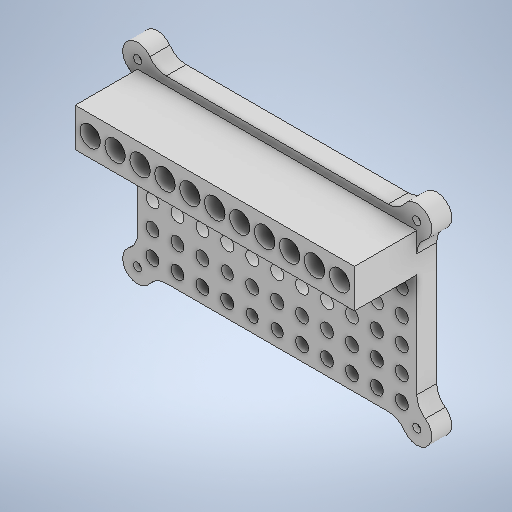
# Autodesk Inventor part: Top_Tip_Matrix
Saved by Autodesk Inventor 2025.2 (Build 292293000, 293)
## iProperties
Created: 2025-02-14
Part Number: Top_Tip_Matrix
Material: Generic
Document SubType Name: Modeling
Designer: m_kni
Density: 1 g/cm^3
Appearance: Default
Author: m_kni
## iProperties of the stored document Top_Tip_Matrix_3DPrint.ipt
Created: 2025-02-16
Part Number: Top_Tip_Matrix_3DPrint
Material: Generic
Document SubType Name: Modeling
Designer: m_kni
Density: 1 g/cm^3
Appearance: Default
Author: m_kni
Autodesk Inventor part; units mm, degrees
ref_plane "YZ Plane" through (0, 0, 0) normal (1, 0, 0) x (0, 1, 0)
ref_plane "XZ Plane" through (0, 0, 0) normal (0, 1, 0) x (-1, 0, 0)
ref_plane "XY Plane" through (0, 0, 0) normal (0, 0, 1) x (1, 0, 0)
sketch "Sketch1" plane through (0, 0, 0) normal (0, 0, 1) x (1, 0, 0)
  line L0 (55, -36) -> (-55, -36)
  line L1 (-55, -36) -> (-55, 36)
  line L2 (-55, 36) -> (55, 36)
  line L3 (55, -36) -> (-55, 36) construction
  line L4 (-55, -36) -> (55, 36) construction
  circle A0 centre (-49, 30) radius 2.425
  circle A1 centre (-49, 20) radius 2.425
  circle A2 centre (-49, 10) radius 2.425
  circle A3 centre (-49, 0) radius 2.425
  circle A4 centre (-49, -10) radius 2.425
  circle A5 centre (-49, -20) radius 2.425
  circle A6 centre (-49, -30) radius 2.425
  circle A7 centre (-39, 30) radius 2.425
  circle A8 centre (-39, 20) radius 2.425
  circle A9 centre (-39, 10) radius 2.425
  circle A10 centre (-39, 0) radius 2.425
  circle A11 centre (-39, -10) radius 2.425
  circle A12 centre (-39, -20) radius 2.425
  circle A13 centre (-39, -30) radius 2.425
  circle A14 centre (-29, 30) radius 2.425
  circle A15 centre (-29, 20) radius 2.425
  circle A16 centre (-29, 10) radius 2.425
  circle A17 centre (-29, 0) radius 2.425
  circle A18 centre (-29, -10) radius 2.425
  circle A19 centre (-29, -20) radius 2.425
  circle A20 centre (-29, -30) radius 2.425
  circle A21 centre (-19, 30) radius 2.425
  circle A22 centre (-19, 20) radius 2.425
  circle A23 centre (-19, 10) radius 2.425
  circle A24 centre (-19, 0) radius 2.425
  circle A25 centre (-19, -10) radius 2.425
  circle A26 centre (-19, -20) radius 2.425
  circle A27 centre (-19, -30) radius 2.425
  circle A28 centre (-9, 30) radius 2.425
  circle A29 centre (-9, 20) radius 2.425
  circle A30 centre (-9, 10) radius 2.425
  circle A31 centre (-9, 0) radius 2.425
  circle A32 centre (-9, -10) radius 2.425
  circle A33 centre (-9, -20) radius 2.425
  circle A34 centre (-9, -30) radius 2.425
  circle A35 centre (1, 30) radius 2.425
  circle A36 centre (1, 20) radius 2.425
  circle A37 centre (1, 10) radius 2.425
  circle A38 centre (1, 0) radius 2.425
  circle A39 centre (1, -10) radius 2.425
  circle A40 centre (1, -20) radius 2.425
  circle A41 centre (1, -30) radius 2.425
  circle A42 centre (11, 30) radius 2.425
  circle A43 centre (11, 20) radius 2.425
  circle A44 centre (11, 10) radius 2.425
  circle A45 centre (11, 0) radius 2.425
  circle A46 centre (11, -10) radius 2.425
  circle A47 centre (11, -20) radius 2.425
  circle A48 centre (11, -30) radius 2.425
  circle A49 centre (21, 30) radius 2.425
  circle A50 centre (21, 20) radius 2.425
  circle A51 centre (21, 10) radius 2.425
  circle A52 centre (21, 0) radius 2.425
  circle A53 centre (21, -10) radius 2.425
  circle A54 centre (21, -20) radius 2.425
  circle A55 centre (21, -30) radius 2.425
  circle A56 centre (31, 30) radius 2.425
  circle A57 centre (31, 20) radius 2.425
  circle A58 centre (31, 10) radius 2.425
  circle A59 centre (31, 0) radius 2.425
  circle A60 centre (31, -10) radius 2.425
  circle A61 centre (31, -20) radius 2.425
  circle A62 centre (31, -30) radius 2.425
  circle A63 centre (41, 30) radius 2.425
  circle A64 centre (41, 20) radius 2.425
  circle A65 centre (41, 10) radius 2.425
  circle A66 centre (41, 0) radius 2.425
  circle A67 centre (41, -10) radius 2.425
  circle A68 centre (41, -20) radius 2.425
  circle A69 centre (41, -30) radius 2.425
  circle A70 centre (51, 30) radius 2.425
  circle A71 centre (51, 20) radius 2.425
  circle A72 centre (51, 10) radius 2.425
  circle A73 centre (51, 0) radius 2.425
  circle A74 centre (51, -10) radius 2.425
  circle A75 centre (51, -20) radius 2.425
  circle A76 centre (51, -30) radius 2.425
  line L5 (-55, 36) -> (57, 36)
  line L6 (57, 36) -> (57, -36)
  line L7 (57, -36) -> (-55, -36)
  line L8 (-55, -36) -> (-55, 36)
  circle A77 centre (-55, 36) radius 6
  circle A78 centre (-55, -36) radius 6
  circle A79 centre (57, 36) radius 6
  circle A80 centre (57, -36) radius 6
  point P0 (0, 0)
  point P1 (57, 30)
  point P2 (-49, -36)
  point P3 (57, -30)
  point P4 (57, 30)
  point P5 (51, 36)
  point P6 (-49, 36)
  point P7 (-55, 30)
  point P8 (-55, -30)
  point P9 (-49, -36)
  point P10 (51, -36)
  dimension "d0" = 110
  dimension "d1" = 72
  dimension "d2" = 4.85
  dimension "d3" = 6
  dimension "d4" = 6
  dimension "d7" = 10
  dimension "d10" = 10
  dimension "d13" = 6
  dimension "d14" = 6
  dimension "d15" = 12
  dimension "d16" = 12
  dimension "d17" = 12
  dimension "d18" = 12
  constraints: 81 centre point, 18 end point, 5 coincident, 3 horizontal, 3 parallel, 2 midpoint, 2 perpendicular, 1 vertical, 152 other
  measures "d0" distance of L1.end L2.end
  measures "d1" distance of L0.end L1.end
  measures "d2" diameter of A0
  measures "d3" distance from line of A0.centre L2
  measures "d4" distance from line of A0.centre L1
  measures "d7" distance of A0.centre A1.centre
  measures "d10" distance of A0.centre A7.centre
  measures "d13" distance of point (57, 30) A70.centre
  measures "d14" distance of point (-49, -36) A6.centre
  measures "d15" diameter of A77
  measures "d16" diameter of A78
  measures "d17" diameter of A79
  measures "d18" diameter of A80
extrude "Extrusion1" add sketch "Sketch1" along normal blind 8
sketch "Sketch2" plane through (0, 0, 8) normal (0, 0, 1) x (1, 0, 0)
  arc A0 (-49, 36) -> (-55, 30) centre (-55, 36) ccw projected
  arc A1 (57, 30) -> (51, 36) centre (57, 36) ccw projected
  line L0 (51, 36) -> (-49, 36) projected
  arc A2 (-49, 36) -> (-55, 30) centre (-55, 36) ccw projected
  line L1 (-55, 30) -> (-55, -30) projected
  arc A3 (-55, -30) -> (-49, -36) centre (-55, -36) ccw projected
  line L2 (-49, -36) -> (51, -36) projected
  arc A4 (51, -36) -> (57, -30) centre (57, -36) ccw projected
  line L3 (57, -30) -> (57, 30) projected
  circle A5 centre (51, -10) radius 2.425 projected
  circle A6 centre (51, 10) radius 2.425 projected
  circle A7 centre (41, -30) radius 2.425 projected
  circle A8 centre (41, -10) radius 2.425 projected
  circle A9 centre (41, 10) radius 2.425 projected
  circle A10 centre (41, 30) radius 2.425 projected
  circle A11 centre (31, -20) radius 2.425 projected
  circle A12 centre (31, 0) radius 2.425 projected
  circle A13 centre (31, 20) radius 2.425 projected
  circle A14 centre (21, -30) radius 2.425 projected
  circle A15 centre (21, -10) radius 2.425 projected
  circle A16 centre (21, 10) radius 2.425 projected
  circle A17 centre (21, 30) radius 2.425 projected
  circle A18 centre (11, -20) radius 2.425 projected
  circle A19 centre (11, 0) radius 2.425 projected
  circle A20 centre (11, 20) radius 2.425 projected
  circle A21 centre (1, -30) radius 2.425 projected
  circle A22 centre (1, -10) radius 2.425 projected
  circle A23 centre (1, 10) radius 2.425 projected
  circle A24 centre (1, 30) radius 2.425 projected
  circle A25 centre (-9, -20) radius 2.425 projected
  circle A26 centre (-9, 0) radius 2.425 projected
  circle A27 centre (-9, 20) radius 2.425 projected
  circle A28 centre (-19, -30) radius 2.425 projected
  circle A29 centre (-19, -10) radius 2.425 projected
  circle A30 centre (-19, 10) radius 2.425 projected
  circle A31 centre (-19, 30) radius 2.425 projected
  circle A32 centre (-29, -20) radius 2.425 projected
  circle A33 centre (-29, 0) radius 2.425 projected
  circle A34 centre (-29, 20) radius 2.425 projected
  circle A35 centre (-39, -30) radius 2.425 projected
  circle A36 centre (-39, -10) radius 2.425 projected
  circle A37 centre (-39, 10) radius 2.425 projected
  circle A38 centre (-49, 20) radius 2.425 projected
  circle A39 centre (-49, 10) radius 2.425 projected
  circle A40 centre (-49, 0) radius 2.425 projected
  circle A41 centre (-49, -10) radius 2.425 projected
  circle A42 centre (-49, -20) radius 2.425 projected
  circle A43 centre (-39, 30) radius 2.425 projected
  circle A44 centre (-39, 20) radius 2.425 projected
  circle A45 centre (-39, 0) radius 2.425 projected
  circle A46 centre (-39, -20) radius 2.425 projected
  circle A47 centre (-29, 30) radius 2.425 projected
  circle A48 centre (-29, 10) radius 2.425 projected
  circle A49 centre (-29, -10) radius 2.425 projected
  circle A50 centre (-29, -30) radius 2.425 projected
  circle A51 centre (-19, 20) radius 2.425 projected
  circle A52 centre (-19, 0) radius 2.425 projected
  circle A53 centre (-19, -20) radius 2.425 projected
  circle A54 centre (-9, 30) radius 2.425 projected
  circle A55 centre (-9, 10) radius 2.425 projected
  circle A56 centre (-9, -10) radius 2.425 projected
  circle A57 centre (-9, -30) radius 2.425 projected
  circle A58 centre (1, 20) radius 2.425 projected
  circle A59 centre (1, 0) radius 2.425 projected
  circle A60 centre (1, -20) radius 2.425 projected
  circle A61 centre (11, 30) radius 2.425 projected
  circle A62 centre (11, 10) radius 2.425 projected
  circle A63 centre (11, -10) radius 2.425 projected
  circle A64 centre (11, -30) radius 2.425 projected
  circle A65 centre (21, 20) radius 2.425 projected
  circle A66 centre (21, 0) radius 2.425 projected
  circle A67 centre (21, -20) radius 2.425 projected
  circle A68 centre (31, 30) radius 2.425 projected
  circle A69 centre (31, 10) radius 2.425 projected
  circle A70 centre (31, -10) radius 2.425 projected
  circle A71 centre (31, -30) radius 2.425 projected
  circle A72 centre (41, 20) radius 2.425 projected
  circle A73 centre (41, 0) radius 2.425 projected
  circle A74 centre (41, -20) radius 2.425 projected
  circle A75 centre (51, 20) radius 2.425 projected
  circle A76 centre (51, 0) radius 2.425 projected
  circle A77 centre (51, -20) radius 2.425 projected
  circle A78 centre (51, -30) radius 2.425 projected
  circle A79 centre (51, 30) radius 2.425 projected
  circle A80 centre (-49, -30) radius 2.425 projected
  circle A81 centre (-49, 30) radius 2.425 projected
  circle A82 centre (-55, 36) radius 4
  circle A83 centre (-55, -36) radius 4
  circle A84 centre (57, -36) radius 4
  circle A85 centre (57, 36) radius 4
  circle A86 centre (-49, 30) radius 2.6
  circle A87 centre (-39, 30) radius 2.6
  circle A88 centre (-29, 30) radius 2.6
  circle A89 centre (-19, 30) radius 2.6
  circle A90 centre (-9, 30) radius 2.6
  circle A91 centre (1, 30) radius 2.6
  circle A92 centre (11, 30) radius 2.6
  circle A93 centre (21, 30) radius 2.6
  circle A94 centre (31, 30) radius 2.6
  circle A95 centre (41, 30) radius 2.6
  circle A96 centre (51, 30) radius 2.6
  circle A97 centre (-49, 20) radius 2.6
  circle A98 centre (-39, 20) radius 2.6
  circle A99 centre (-29, 20) radius 2.6
  circle A100 centre (-19, 20) radius 2.6
  circle A101 centre (-9, 20) radius 2.6
  circle A102 centre (1, 20) radius 2.6
  circle A103 centre (11, 20) radius 2.6
  circle A104 centre (21, 20) radius 2.6
  circle A105 centre (31, 20) radius 2.6
  circle A106 centre (41, 20) radius 2.6
  circle A107 centre (51, 20) radius 2.6
  circle A108 centre (-49, 10) radius 2.6
  circle A109 centre (-39, 10) radius 2.6
  circle A110 centre (-29, 10) radius 2.6
  circle A111 centre (-19, 10) radius 2.6
  circle A112 centre (-9, 10) radius 2.6
  circle A113 centre (1, 10) radius 2.6
  circle A114 centre (11, 10) radius 2.6
  circle A115 centre (21, 10) radius 2.6
  circle A116 centre (31, 10) radius 2.6
  circle A117 centre (41, 10) radius 2.6
  circle A118 centre (51, 10) radius 2.6
  circle A119 centre (-49, 0) radius 2.6
  circle A120 centre (-39, 0) radius 2.6
  circle A121 centre (-29, 0) radius 2.6
  circle A122 centre (-19, 0) radius 2.6
  circle A123 centre (-9, 0) radius 2.6
  circle A124 centre (1, 0) radius 2.6
  circle A125 centre (11, 0) radius 2.6
  circle A126 centre (21, 0) radius 2.6
  circle A127 centre (31, 0) radius 2.6
  circle A128 centre (41, 0) radius 2.6
  circle A129 centre (51, 0) radius 2.6
  circle A130 centre (-49, -10) radius 2.6
  circle A131 centre (-39, -10) radius 2.6
  circle A132 centre (-29, -10) radius 2.6
  circle A133 centre (-19, -10) radius 2.6
  circle A134 centre (-9, -10) radius 2.6
  circle A135 centre (1, -10) radius 2.6
  circle A136 centre (11, -10) radius 2.6
  circle A137 centre (21, -10) radius 2.6
  circle A138 centre (31, -10) radius 2.6
  circle A139 centre (41, -10) radius 2.6
  circle A140 centre (51, -10) radius 2.6
  circle A141 centre (-49, -20) radius 2.6
  circle A142 centre (-39, -20) radius 2.6
  circle A143 centre (-29, -20) radius 2.6
  circle A144 centre (-19, -20) radius 2.6
  circle A145 centre (-9, -20) radius 2.6
  circle A146 centre (1, -20) radius 2.6
  circle A147 centre (11, -20) radius 2.6
  circle A148 centre (21, -20) radius 2.6
  circle A149 centre (31, -20) radius 2.6
  circle A150 centre (41, -20) radius 2.6
  circle A151 centre (51, -20) radius 2.6
  circle A152 centre (-49, -30) radius 2.6
  circle A153 centre (-39, -30) radius 2.6
  circle A154 centre (-29, -30) radius 2.6
  circle A155 centre (-19, -30) radius 2.6
  circle A156 centre (-9, -30) radius 2.6
  circle A157 centre (1, -30) radius 2.6
  circle A158 centre (11, -30) radius 2.6
  circle A159 centre (21, -30) radius 2.6
  circle A160 centre (31, -30) radius 2.6
  circle A161 centre (41, -30) radius 2.6
  circle A162 centre (51, -30) radius 2.6
  point P0 (0, 0)
  dimension "d21" = 8
  dimension "d22" = 8
  dimension "d23" = 8
  dimension "d24" = 8
  dimension "d36" = 4.85
  dimension "d37" = 5.2
  dimension "d40" = 10
  dimension "d43" = 10
  constraints: 81 centre point, 5 coincident, 1 horizontal, 1 vertical, 152 other
  measures "d21" diameter of A82
  measures "d22" diameter of A83
  measures "d23" diameter of A84
  measures "d24" diameter of A85
  measures "d36" diameter of A64
  measures "d37" diameter of A86
  measures "d40" distance of A86.centre A87.centre
  measures "d43" distance of A86.centre A97.centre
extrude "Extrusion2" cut sketch "Sketch2" against normal blind 8 contours A82 | A83 | A84 | A85
sketch "Sketch3" plane through (0, 0, 8) normal (0, 0, 1) x (1, 0, 0)
  circle A0 centre (-55, 36) radius 4 projected
  circle A1 centre (-55, -36) radius 4 projected
  circle A2 centre (57, 36) radius 4 projected
  circle A3 centre (57, -36) radius 4 projected
  point P0 (0, 0)
extrude "Extrusion3" add sketch "Sketch3" against normal blind 2
sketch "Sketch4" plane through (0, 0, 8) normal (0, 0, 1) x (1, 0, 0)
  arc A0 (-49, 36) -> (-55, 30) centre (-55, 36) ccw projected
  arc A1 (57, 30) -> (51, 36) centre (57, 36) ccw projected
  arc A2 (-55, -30) -> (-49, -36) centre (-55, -36) ccw projected
  arc A3 (51, -36) -> (57, -30) centre (57, -36) ccw projected
  circle A4 centre (-55, 36) radius 1.6
  circle A5 centre (-55, -36) radius 4 projected
  circle A6 centre (-55, -36) radius 1.6
  circle A7 centre (57, 36) radius 1.6
  circle A8 centre (57, -36) radius 1.6
  point P0 (0, 0)
  dimension "d29" = 3.2
  dimension "d30" = 3.2
  dimension "d31" = 3.2
  dimension "d32" = 3.2
  constraints: 4 centre point, 4 coincident
  measures "d29" diameter of A4
  measures "d30" diameter of A6
  measures "d31" diameter of A7
  measures "d32" diameter of A8
extrude "Extrusion4" cut sketch "Sketch4" against normal blind 22.6375 contours A4 | A6 | A7 | A8
fillet "Fillet1" radius 8 8 edges at (-49, 36, 4) (51, 36, 4) (57, 30, 4) (57, -30, 4) (51, -36, 4) (-49, -36, 4) (-55, -30, 4) (-55, 30, 4)
sketch "Sketch5" plane through (0, 0, 0) normal (0, 0, -1) x (-1, 0, 0)
  circle A0 centre (49, 30) radius 2.425 projected
  circle A1 centre (39, 30) radius 2.425 projected
  circle A2 centre (-57, -36) radius 4 projected
  circle A3 centre (55, -36) radius 4 projected
  circle A4 centre (-57, 36) radius 4 projected
  circle A5 centre (55, 36) radius 4 projected
  arc A6 (-57, 24.5109) -> (-60.4286, 31.0761) centre (-65, 24.5109) ccw projected
  line L0 (-57, -24.5109) -> (-57, 24.5109) projected
  arc A7 (-60.4286, -31.0761) -> (-57, -24.5109) centre (-65, -24.5109) ccw projected
  arc A8 (-60.4286, -31.0761) -> (-52.0761, -39.4286) centre (-57, -36) ccw projected
  arc A9 (-45.5109, -36) -> (-52.0761, -39.4286) centre (-45.5109, -44) ccw projected
  line L1 (43.5109, -36) -> (-45.5109, -36) projected
  arc A10 (50.0761, -39.4286) -> (43.5109, -36) centre (43.5109, -44) ccw projected
  arc A11 (50.0761, -39.4286) -> (58.4286, -31.0761) centre (55, -36) ccw projected
  arc A12 (55, -24.5109) -> (58.4286, -31.0761) centre (63, -24.5109) ccw projected
  line L2 (55, 24.5109) -> (55, -24.5109) projected
  arc A13 (58.4286, 31.0761) -> (55, 24.5109) centre (63, 24.5109) ccw projected
  arc A14 (58.4286, 31.0761) -> (50.0761, 39.4286) centre (55, 36) ccw projected
  arc A15 (43.5109, 36) -> (50.0761, 39.4286) centre (43.5109, 44) ccw projected
  line L3 (-45.5109, 36) -> (43.5109, 36) projected
  arc A16 (-52.0761, 39.4286) -> (-45.5109, 36) centre (-45.5109, 44) ccw projected
  arc A17 (-52.0761, 39.4286) -> (-60.4286, 31.0761) centre (-57, 36) ccw projected
  circle A18 centre (-51, -10) radius 2.425 projected
  circle A19 centre (-51, 10) radius 2.425 projected
  circle A20 centre (-41, -30) radius 2.425 projected
  circle A21 centre (-41, -10) radius 2.425 projected
  circle A22 centre (-41, 10) radius 2.425 projected
  circle A23 centre (-41, 30) radius 2.425 projected
  circle A24 centre (-31, -20) radius 2.425 projected
  circle A25 centre (-31, 0) radius 2.425 projected
  circle A26 centre (-31, 20) radius 2.425 projected
  circle A27 centre (-21, -30) radius 2.425 projected
  circle A28 centre (-21, -10) radius 2.425 projected
  circle A29 centre (-21, 10) radius 2.425 projected
  circle A30 centre (-21, 30) radius 2.425 projected
  circle A31 centre (-11, -20) radius 2.425 projected
  circle A32 centre (-11, 0) radius 2.425 projected
  circle A33 centre (-11, 20) radius 2.425 projected
  circle A34 centre (-1, -30) radius 2.425 projected
  circle A35 centre (-1, -10) radius 2.425 projected
  circle A36 centre (-1, 10) radius 2.425 projected
  circle A37 centre (-1, 30) radius 2.425 projected
  circle A38 centre (9, -20) radius 2.425 projected
  circle A39 centre (9, 0) radius 2.425 projected
  circle A40 centre (9, 20) radius 2.425 projected
  circle A41 centre (19, -30) radius 2.425 projected
  circle A42 centre (19, -10) radius 2.425 projected
  circle A43 centre (19, 10) radius 2.425 projected
  circle A44 centre (19, 30) radius 2.425 projected
  circle A45 centre (29, -20) radius 2.425 projected
  circle A46 centre (29, 0) radius 2.425 projected
  circle A47 centre (29, 20) radius 2.425 projected
  circle A48 centre (39, -30) radius 2.425 projected
  circle A49 centre (39, -10) radius 2.425 projected
  circle A50 centre (39, 10) radius 2.425 projected
  circle A51 centre (49, 20) radius 2.425 projected
  circle A52 centre (49, 10) radius 2.425 projected
  circle A53 centre (49, 0) radius 2.425 projected
  circle A54 centre (49, -10) radius 2.425 projected
  circle A55 centre (49, -20) radius 2.425 projected
  circle A56 centre (39, 30) radius 2.425 projected
  circle A57 centre (39, 20) radius 2.425 projected
  circle A58 centre (39, 0) radius 2.425 projected
  circle A59 centre (39, -20) radius 2.425 projected
  circle A60 centre (29, 30) radius 2.425 projected
  circle A61 centre (29, 10) radius 2.425 projected
  circle A62 centre (29, -10) radius 2.425 projected
  circle A63 centre (29, -30) radius 2.425 projected
  circle A64 centre (19, 20) radius 2.425 projected
  circle A65 centre (19, 0) radius 2.425 projected
  circle A66 centre (19, -20) radius 2.425 projected
  circle A67 centre (9, 30) radius 2.425 projected
  circle A68 centre (9, 10) radius 2.425 projected
  circle A69 centre (9, -10) radius 2.425 projected
  circle A70 centre (9, -30) radius 2.425 projected
  circle A71 centre (-1, 20) radius 2.425 projected
  circle A72 centre (-1, 0) radius 2.425 projected
  circle A73 centre (-1, -20) radius 2.425 projected
  circle A74 centre (-11, 30) radius 2.425 projected
  circle A75 centre (-11, 10) radius 2.425 projected
  circle A76 centre (-11, -10) radius 2.425 projected
  circle A77 centre (-11, -30) radius 2.425 projected
  circle A78 centre (-21, 20) radius 2.425 projected
  circle A79 centre (-21, 0) radius 2.425 projected
  circle A80 centre (-21, -20) radius 2.425 projected
  circle A81 centre (-31, 30) radius 2.425 projected
  circle A82 centre (-31, 10) radius 2.425 projected
  circle A83 centre (-31, -10) radius 2.425 projected
  circle A84 centre (-31, -30) radius 2.425 projected
  circle A85 centre (-41, 20) radius 2.425 projected
  circle A86 centre (-41, 0) radius 2.425 projected
  circle A87 centre (-41, -20) radius 2.425 projected
  circle A88 centre (-51, 20) radius 2.425 projected
  circle A89 centre (-51, 0) radius 2.425 projected
  circle A90 centre (-51, -20) radius 2.425 projected
  circle A91 centre (-51, -30) radius 2.425 projected
  circle A92 centre (-51, 30) radius 2.425 projected
  circle A93 centre (49, -30) radius 2.425 projected
  circle A94 centre (49, 30) radius 2.425 projected
  circle A95 centre (29, 30) radius 2.425 projected
  circle A96 centre (49, 30) radius 2.625
  circle A97 centre (49, 20) radius 2.625
  circle A98 centre (49, 10) radius 2.625
  circle A99 centre (49, 0) radius 2.625
  circle A100 centre (49, -10) radius 2.625
  circle A101 centre (49, -20) radius 2.625
  circle A102 centre (49, -30) radius 2.625
  circle A103 centre (39, 30) radius 2.625
  circle A104 centre (39, 20) radius 2.625
  circle A105 centre (39, 10) radius 2.625
  circle A106 centre (39, 0) radius 2.625
  circle A107 centre (39, -10) radius 2.625
  circle A108 centre (39, -20) radius 2.625
  circle A109 centre (39, -30) radius 2.625
  circle A110 centre (29, 30) radius 2.625
  circle A111 centre (29, 20) radius 2.625
  circle A112 centre (29, 10) radius 2.625
  circle A113 centre (29, 0) radius 2.625
  circle A114 centre (29, -10) radius 2.625
  circle A115 centre (29, -20) radius 2.625
  circle A116 centre (29, -30) radius 2.625
  circle A117 centre (19, 30) radius 2.625
  circle A118 centre (19, 20) radius 2.625
  circle A119 centre (19, 10) radius 2.625
  circle A120 centre (19, 0) radius 2.625
  circle A121 centre (19, -10) radius 2.625
  circle A122 centre (19, -20) radius 2.625
  circle A123 centre (19, -30) radius 2.625
  circle A124 centre (9, 30) radius 2.625
  circle A125 centre (9, 20) radius 2.625
  circle A126 centre (9, 10) radius 2.625
  circle A127 centre (9, 0) radius 2.625
  circle A128 centre (9, -10) radius 2.625
  circle A129 centre (9, -20) radius 2.625
  circle A130 centre (9, -30) radius 2.625
  circle A131 centre (-1, 30) radius 2.625
  circle A132 centre (-1, 20) radius 2.625
  circle A133 centre (-1, 10) radius 2.625
  circle A134 centre (-1, 0) radius 2.625
  circle A135 centre (-1, -10) radius 2.625
  circle A136 centre (-1, -20) radius 2.625
  circle A137 centre (-1, -30) radius 2.625
  circle A138 centre (-11, 30) radius 2.625
  circle A139 centre (-11, 20) radius 2.625
  circle A140 centre (-11, 10) radius 2.625
  circle A141 centre (-11, 0) radius 2.625
  circle A142 centre (-11, -10) radius 2.625
  circle A143 centre (-11, -20) radius 2.625
  circle A144 centre (-11, -30) radius 2.625
  circle A145 centre (-21, 30) radius 2.625
  circle A146 centre (-21, 20) radius 2.625
  circle A147 centre (-21, 10) radius 2.625
  circle A148 centre (-21, 0) radius 2.625
  circle A149 centre (-21, -10) radius 2.625
  circle A150 centre (-21, -20) radius 2.625
  circle A151 centre (-21, -30) radius 2.625
  circle A152 centre (-31, 30) radius 2.625
  circle A153 centre (-31, 20) radius 2.625
  circle A154 centre (-31, 10) radius 2.625
  circle A155 centre (-31, 0) radius 2.625
  circle A156 centre (-31, -10) radius 2.625
  circle A157 centre (-31, -20) radius 2.625
  circle A158 centre (-31, -30) radius 2.625
  circle A159 centre (-41, 30) radius 2.625
  circle A160 centre (-41, 20) radius 2.625
  circle A161 centre (-41, 10) radius 2.625
  circle A162 centre (-41, 0) radius 2.625
  circle A163 centre (-41, -10) radius 2.625
  circle A164 centre (-41, -20) radius 2.625
  circle A165 centre (-41, -30) radius 2.625
  circle A166 centre (-51, 30) radius 2.625
  circle A167 centre (-51, 20) radius 2.625
  circle A168 centre (-51, 10) radius 2.625
  circle A169 centre (-51, 0) radius 2.625
  circle A170 centre (-51, -10) radius 2.625
  circle A171 centre (-51, -20) radius 2.625
  circle A172 centre (-51, -30) radius 2.625
  point P0 (0, 0)
  dimension "d46" = 5.25
  dimension "d49" = 10
  dimension "d52" = 10
  constraints: 77 centre point, 1 coincident, 1 horizontal, 1 vertical, 152 other
  measures "d46" diameter of A96
  measures "d49" distance of A96.centre A97.centre
  measures "d52" distance of A96.centre A103.centre
extrude "Extrusion5" cut sketch "Sketch5" against normal blind 10 contours A0 | A1 | A18 | A19 | A20 | A21 | A22 | A23 | A24 | A25 | A26 | A27 | A28 | A29 | A30 | A31 | A32 | A33 | A34 | A35 | A36 | A37 | A38 | A39 | A40 | A41 | A42 | A43 | A44 | A45 | A46 | A47 | A48 | A49 | A50 | A51 | A52 | A53 | A54 | A55 | A57 | A58 | A59 | A60 | A61 | A62 | A63 | A64 | A65 | A66 | A67 | A68 | A69 | A70 | A71 | A72 | A73 | A74 | A75 | A76 | A77 | A78 | A79 | A80 | A81 | A82 | A83 | A84 | A85 | A86 | A87 | A88 | A89 | A90 | A91 | A92 | A93 | A96 | A97 | A98 | A99 | A100 | A101 | A102 | A103 | A104 | A105 | A106 | A107 | A108 | A109 | A110 | A111 | A112 | A113 | A114 | A115 | A116 | A117 | A118 | A119 | A120 | A121 | A123 | A124 | A125 | A126 | A127 | A128 | A129 | A131 | A132 | A133 | A134 | A135 | A136 | A138 | A139 | A140 | A141 | A142 | A143 | A144 | A145 | A146 | A147 | A148 | A149 | A150 | A151 | A152 | A153 | A154 | A155 | A156 | A157 | A158 | A159 | A160 | A161 | A162 | A163 | A164 | A165 | A166 | A167 | A168 | A169 | A170 | A171 | A172
sketch "Sketch7" plane through (0, 0, 8) normal (0, 0, 1) x (1, 0, 0)
  line L0 (-55, 24.5109) -> (-55, -24.5109) projected
  line L1 (-55, 17.1851) -> (57, 17.1851)
  line L2 (57, -24.5109) -> (57, 24.5109) projected
  line L3 (-55, 17.1851) -> (53.625, 17.1851)
  line L4 (53.625, 17.1851) -> (53.625, 32.625)
  line L5 (53.625, 32.625) -> (-55, 32.625)
  line L6 (-55, 32.625) -> (-55, 17.1851)
  line L7 (57, 17.1851) -> (57, 32.625)
  line L8 (57, 32.625) -> (53.625, 32.625)
  point P0 (0, 0)
  constraints: 14 end point, 2 horizontal, 2 parallel, 2 perpendicular, 2 point on line, 1 vertical
extrude "Extrusion6" add sketch "Sketch7" along normal blind 25
sketch "Sketch8" plane through (0, 0, 33) normal (0, 0, 1) x (1, 0, 0)
  line L0 (-55, 32.625) -> (-55, 17.1851) projected
  line L1 (-55, 24.905) -> (57, 24.905)
  line L2 (57, 17.1851) -> (57, 32.625) projected
  circle A0 centre (-49, 24.905) radius 4.1
  circle A1 centre (-39, 24.905) radius 4.1
  circle A2 centre (-29, 24.905) radius 4.1
  circle A3 centre (-19, 24.905) radius 4.1
  circle A4 centre (-9, 24.905) radius 4.1
  circle A5 centre (1, 24.905) radius 4.1
  circle A6 centre (11, 24.905) radius 4.1
  circle A7 centre (21, 24.905) radius 4.1
  circle A8 centre (31, 24.905) radius 4.1
  circle A9 centre (41, 24.905) radius 4.1
  circle A10 centre (51, 24.905) radius 4.1
  point P0 (0, 0)
  dimension "d59" = 8.2
  dimension "d60" = 6
  dimension "d63" = 10
  constraints: 11 centre point, 2 end point, 2 midpoint, 1 horizontal, 1 point on line, 20 other
  measures "d59" diameter of A0
  measures "d60" distance from line of L0 A0.centre
  measures "d63" distance of A0.centre A1.centre
extrude "Extrusion7" cut sketch "Sketch8" against normal blind 40.875
sketch "Sketch9" plane through (0, 0, 0) normal (0, 0, -1) x (-1, 0, 0)
  arc A0 (31.1939, 21.4414) -> (31.1007, 28.426) centre (29, 24.905) ccw projected
  arc A1 (26.8061, 21.4414) -> (31.1939, 21.4414) centre (29, 20) ccw projected
  arc A2 (26.8993, 28.426) -> (26.8061, 21.4414) centre (29, 24.905) ccw projected
  arc A3 (31.1007, 28.426) -> (26.8993, 28.426) centre (29, 30) ccw projected
  arc A4 (-8.8061, 21.4414) -> (-8.8993, 28.426) centre (-11, 24.905) ccw projected
  arc A5 (-13.1939, 21.4414) -> (-8.8061, 21.4414) centre (-11, 20) ccw projected
  arc A6 (-13.1007, 28.426) -> (-13.1939, 21.4414) centre (-11, 24.905) ccw projected
  arc A7 (-8.8993, 28.426) -> (-13.1007, 28.426) centre (-11, 30) ccw projected
  arc A8 (-48.8061, 21.4414) -> (-48.8993, 28.426) centre (-51, 24.905) ccw projected
  arc A9 (-53.1939, 21.4414) -> (-48.8061, 21.4414) centre (-51, 20) ccw projected
  arc A10 (-53.1007, 28.426) -> (-53.1939, 21.4414) centre (-51, 24.905) ccw projected
  arc A11 (-48.8993, 28.426) -> (-53.1007, 28.426) centre (-51, 30) ccw projected
  arc A12 (-18.8061, 21.4414) -> (-18.8993, 28.426) centre (-21, 24.905) ccw projected
  arc A13 (-23.1939, 21.4414) -> (-18.8061, 21.4414) centre (-21, 20) ccw projected
  arc A14 (-23.1007, 28.426) -> (-23.1939, 21.4414) centre (-21, 24.905) ccw projected
  arc A15 (-18.8993, 28.426) -> (-23.1007, 28.426) centre (-21, 30) ccw projected
  arc A16 (21.1939, 21.4414) -> (21.1007, 28.426) centre (19, 24.905) ccw projected
  arc A17 (16.8061, 21.4414) -> (21.1939, 21.4414) centre (19, 20) ccw projected
  arc A18 (16.8993, 28.426) -> (16.8061, 21.4414) centre (19, 24.905) ccw projected
  arc A19 (21.1007, 28.426) -> (16.8993, 28.426) centre (19, 30) ccw projected
  arc A20 (41.1939, 21.4414) -> (41.1007, 28.426) centre (39, 24.905) ccw projected
  arc A21 (36.8061, 21.4414) -> (41.1939, 21.4414) centre (39, 20) ccw projected
  arc A22 (36.8993, 28.426) -> (36.8061, 21.4414) centre (39, 24.905) ccw projected
  arc A23 (41.1007, 28.426) -> (36.8993, 28.426) centre (39, 30) ccw projected
  arc A24 (1.1939, 21.4414) -> (1.1007, 28.426) centre (-1, 24.905) ccw projected
  arc A25 (-3.1939, 21.4414) -> (1.1939, 21.4414) centre (-1, 20) ccw projected
  arc A26 (-3.1007, 28.426) -> (-3.1939, 21.4414) centre (-1, 24.905) ccw projected
  arc A27 (1.1007, 28.426) -> (-3.1007, 28.426) centre (-1, 30) ccw projected
  arc A28 (-38.8061, 21.4414) -> (-38.8993, 28.426) centre (-41, 24.905) ccw projected
  arc A29 (-43.1939, 21.4414) -> (-38.8061, 21.4414) centre (-41, 20) ccw projected
  arc A30 (-43.1007, 28.426) -> (-43.1939, 21.4414) centre (-41, 24.905) ccw projected
  arc A31 (-38.8993, 28.426) -> (-43.1007, 28.426) centre (-41, 30) ccw projected
  arc A32 (-28.8061, 21.4414) -> (-28.8993, 28.426) centre (-31, 24.905) ccw projected
  arc A33 (-33.1939, 21.4414) -> (-28.8061, 21.4414) centre (-31, 20) ccw projected
  arc A34 (-33.1007, 28.426) -> (-33.1939, 21.4414) centre (-31, 24.905) ccw projected
  arc A35 (-28.8993, 28.426) -> (-33.1007, 28.426) centre (-31, 30) ccw projected
  arc A36 (11.1939, 21.4414) -> (11.1007, 28.426) centre (9, 24.905) ccw projected
  arc A37 (6.8061, 21.4414) -> (11.1939, 21.4414) centre (9, 20) ccw projected
  arc A38 (6.8993, 28.426) -> (6.8061, 21.4414) centre (9, 24.905) ccw projected
  arc A39 (11.1007, 28.426) -> (6.8993, 28.426) centre (9, 30) ccw projected
  arc A40 (51.1939, 21.4414) -> (51.1007, 28.426) centre (49, 24.905) ccw projected
  arc A41 (46.8061, 21.4414) -> (51.1939, 21.4414) centre (49, 20) ccw projected
  arc A42 (46.8993, 28.426) -> (46.8061, 21.4414) centre (49, 24.905) ccw projected
  arc A43 (51.1007, 28.426) -> (46.8993, 28.426) centre (49, 30) ccw projected
  circle A44 centre (49, 10) radius 2.625 projected
  circle A45 centre (-51, -10) radius 2.625 projected
  circle A46 centre (-41, -30) radius 2.625 projected
  circle A47 centre (-31, -10) radius 2.625 projected
  circle A48 centre (-31, -30) radius 2.625 projected
  circle A49 centre (-11, 0) radius 2.625 projected
  circle A50 centre (-11, 10) radius 2.625 projected
  circle A51 centre (-1, 0) radius 2.625 projected
  circle A52 centre (49, -10) radius 2.625 projected
  circle A53 centre (39, -20) radius 2.625 projected
  circle A54 centre (29, -30) radius 2.625 projected
  circle A55 centre (19, 10) radius 2.625 projected
  circle A56 centre (19, -30) radius 2.625 projected
  circle A57 centre (9, 0) radius 2.625 projected
  circle A58 centre (19, 0) radius 2.625 projected
  circle A59 centre (29, -10) radius 2.625 projected
  circle A60 centre (39, -10) radius 2.625 projected
  circle A61 centre (49, -20) radius 2.625 projected
  circle A62 centre (9, -20) radius 2.625 projected
  circle A63 centre (-1, -10) radius 2.625 projected
  circle A64 centre (-1, 10) radius 2.625 projected
  circle A65 centre (-11, -30) radius 2.625 projected
  circle A66 centre (-31, -20) radius 2.625 projected
  circle A67 centre (-21, -10) radius 2.625 projected
  circle A68 centre (-41, 0) radius 2.625 projected
  circle A69 centre (-51, 0) radius 2.625 projected
  circle A70 centre (39, 10) radius 2.625 projected
  circle A71 centre (-51, -20) radius 2.625 projected
  circle A72 centre (-41, -20) radius 2.625 projected
  circle A73 centre (-51, 10) radius 2.625 projected
  circle A74 centre (-31, 0) radius 2.625 projected
  circle A75 centre (-21, 10) radius 2.625 projected
  circle A76 centre (-21, -30) radius 2.625 projected
  circle A77 centre (-11, -10) radius 2.625 projected
  circle A78 centre (49, 0) radius 2.625 projected
  circle A79 centre (39, -30) radius 2.625 projected
  circle A80 centre (29, -20) radius 2.625 projected
  circle A81 centre (29, 10) radius 2.625 projected
  circle A82 centre (9, 10) radius 2.625 projected
  circle A83 centre (19, -10) radius 2.625 projected
  circle A84 centre (29, 0) radius 2.625 projected
  circle A85 centre (39, 0) radius 2.625 projected
  circle A86 centre (49, -30) radius 2.625 projected
  circle A87 centre (9, -10) radius 2.625 projected
  circle A88 centre (-1, -20) radius 2.625 projected
  circle A89 centre (-11, -20) radius 2.625 projected
  circle A90 centre (-21, -20) radius 2.625 projected
  circle A91 centre (-21, 0) radius 2.625 projected
  circle A92 centre (-31, 10) radius 2.625 projected
  circle A93 centre (-41, 10) radius 2.625 projected
  circle A94 centre (-41, -10) radius 2.625 projected
  circle A95 centre (-51, -30) radius 2.625 projected
  circle A96 centre (-57, -36) radius 4 projected
  circle A97 centre (55, -36) radius 4 projected
  circle A98 centre (-57, 36) radius 4 projected
  circle A99 centre (55, 36) radius 4 projected
  arc A100 (-57, 24.5109) -> (-60.4286, 31.0761) centre (-65, 24.5109) ccw projected
  line L0 (-57, -24.5109) -> (-57, 24.5109) projected
  arc A101 (-60.4286, -31.0761) -> (-57, -24.5109) centre (-65, -24.5109) ccw projected
  arc A102 (-60.4286, -31.0761) -> (-52.0761, -39.4286) centre (-57, -36) ccw projected
  arc A103 (-45.5109, -36) -> (-52.0761, -39.4286) centre (-45.5109, -44) ccw projected
  line L1 (43.5109, -36) -> (-45.5109, -36) projected
  arc A104 (50.0761, -39.4286) -> (43.5109, -36) centre (43.5109, -44) ccw projected
  arc A105 (50.0761, -39.4286) -> (58.4286, -31.0761) centre (55, -36) ccw projected
  arc A106 (55, -24.5109) -> (58.4286, -31.0761) centre (63, -24.5109) ccw projected
  line L2 (55, 24.5109) -> (55, -24.5109) projected
  arc A107 (58.4286, 31.0761) -> (55, 24.5109) centre (63, 24.5109) ccw projected
  arc A108 (58.4286, 31.0761) -> (50.0761, 39.4286) centre (55, 36) ccw projected
  arc A109 (43.5109, 36) -> (50.0761, 39.4286) centre (43.5109, 44) ccw projected
  line L3 (-45.5109, 36) -> (43.5109, 36) projected
  arc A110 (-52.0761, 39.4286) -> (-45.5109, 36) centre (-45.5109, 44) ccw projected
  arc A111 (-52.0761, 39.4286) -> (-60.4286, 31.0761) centre (-57, 36) ccw projected
  circle A112 centre (-1, -30) radius 2.425 projected
  circle A113 centre (19, -20) radius 2.425 projected
  circle A114 centre (9, -30) radius 2.425 projected
  circle A115 centre (-51, 24.905) radius 4.1
  circle A116 centre (-41, 24.905) radius 4.1
  circle A117 centre (-31, 24.905) radius 4.1
  circle A118 centre (-21, 24.905) radius 4.1
  circle A119 centre (-11, 24.905) radius 4.1
  circle A120 centre (-1, 24.905) radius 4.1
  circle A121 centre (9, 24.905) radius 4.1
  circle A122 centre (19, 24.905) radius 4.1
  circle A123 centre (29, 24.905) radius 4.1
  circle A124 centre (39, 24.905) radius 4.1
  circle A125 centre (49, 24.905) radius 4.1
  point P0 (0, 0)
  point P1 (51.1939, 21.4414)
  point P2 (46.8993, 28.426)
  point P3 (36.8993, 28.426)
  point P4 (41.1939, 21.4414)
  point P5 (36.8061, 21.4414)
  point P6 (26.8993, 28.426)
  point P7 (31.1007, 28.426)
  point P8 (16.8993, 28.426)
  point P9 (21.1007, 28.426)
  point P10 (11.1939, 21.4414)
  point P11 (6.8061, 21.4414)
  point P12 (6.8993, 28.426)
  point P13 (11.1007, 28.426)
  point P14 (-3.1007, 28.426)
  point P15 (1.1007, 28.426)
  point P16 (1.1939, 21.4414)
  point P17 (-3.1939, 21.4414)
  point P18 (-13.1007, 28.426)
  point P19 (-8.8061, 21.4414)
  point P20 (-18.8061, 21.4414)
  point P21 (-28.8061, 21.4414)
  point P22 (-38.8061, 21.4414)
  point P23 (-43.1007, 28.426)
  point P24 (-53.1007, 28.426)
  point P25 (-48.8061, 21.4414)
  constraints: 11 centre point, 11 coincident, 7 concentric
extrude "Extrusion8" add sketch "Sketch9" against normal up to surface (33 mm away) contours A1 A123 | A123 A3 | A5 A119 | A119 A7 | A9 A115 | A115 A11 | A13 A118 | A118 A15 | A17 A122 | A122 A19 | A21 A124 | A124 A23 | A25 A120 | A120 A27 | A29 A116 | A116 A31 | A33 A117 | A117 A35 | A37 A121 | A121 A39 | A41 A125 | A125 A43
body "Solid1"
